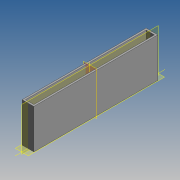
# Autodesk Inventor part: P024_ReservoirSilica
Saved by Autodesk Inventor 2021.3 (Build 253353000, 353)
## iProperties
Created: 2021-11-19
Part Number: P024_ReservoirSilica
Material: Générique
Document SubType Name: Modeling
Designer: gabri
Density: 1 g/cm^3
Appearance: Par défaut
Author: gabri
Autodesk Inventor part; units mm, degrees
sketch "Sketch4" plane through (0, 0, 0) normal (0, 0, 1) x (1, 0, 0)
  line L0 (-7, -74) -> (7, -74)
  line L1 (7, -74) -> (7, 74)
  line L2 (7, 74) -> (-7, 74)
  line L3 (-7, 74) -> (-7, -74)
  line L4 (-7, -74) -> (7, 74) construction
  line L5 (7, -74) -> (-7, 74) construction
  line L6 (-5, 72) -> (5, 72)
  line L7 (5, 72) -> (5, -72)
  line L8 (5, -72) -> (-5, -72)
  line L9 (-5, -72) -> (-5, 72)
  line L10 (-5, 72) -> (5, -72) construction
  line L11 (5, 72) -> (-5, -72) construction
  point P0 (0, 0)
  dimension "d6" = 148
  dimension "d7" = 14
  dimension "d10" = 2
  dimension "d11" = 2
  constraints: 24 end point, 4 midpoint, 4 parallel, 2 horizontal, 2 perpendicular
  measures "d6" distance of L0.end L1.end
  measures "d7" distance of L1.end L2.end
  measures "d10" distance between parallel lines of L0 L8
  measures "d11" distance between parallel lines of L3 L9
extrude "Extrusion1" add sketch "Sketch4" along normal blind 47
body "Solid2"
